# Autodesk Inventor part: M04POLAR
Saved by Autodesk Inventor 2013 (Build 170138000, 138)
## iProperties
Created: 2014-11-03
Part Number: M04POLAR
Material: Generic
Document SubType Name: Modeling
Designer: Jeramy
Density: 1 g/cm^3
Author: Jeramy
Autodesk Inventor part; units mm, degrees
ref_plane "YZ Plane" through (0, 0, 0) normal (1, 0, 0) x (0, 1, 0)
ref_plane "XZ Plane" through (0, 0, 0) normal (0, 1, 0) x (-1, 0, 0)
ref_plane "XY Plane" through (0, 0, 0) normal (0, 0, 1) x (1, 0, 0)
sketch "MOLEX-1X4, M04POLAR_1" plane through (0, 0, 0) normal (0, 0, 1) x (1, 0, 0)
  line L0 (-1.3, -2.5) -> (-1.3, 3)
  line L1 (-1.3, 3) -> (8.9, 3)
  line L2 (8.9, 3) -> (8.9, -2.5)
  line L3 (8.9, -2.5) -> (-1.3, -2.5)
  constraints: 8 end point
extrude "Extrusion1" add sketch "MOLEX-1X4, M04POLAR_1" along normal blind 0.01
body "Solid1"
